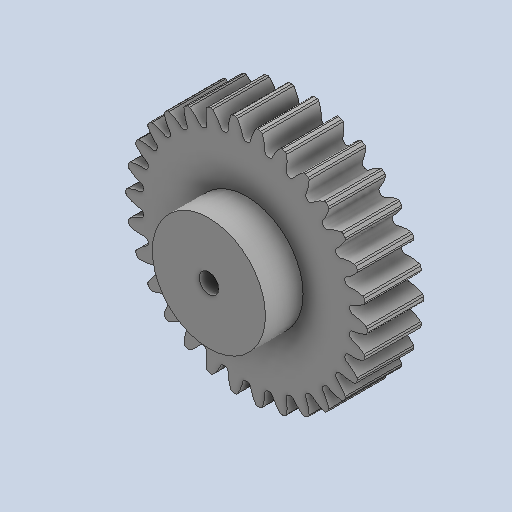
# Autodesk Inventor part: input_gear_3
Saved by Autodesk Inventor 2024 (Build 280153000, 153)
## iProperties
Created: 2023-10-31
Part Number: input_gear_3
Material: Generic
Document SubType Name: Modeling
Designer: MATEO
Density: 1 g/cm^3
Appearance: Default
Mass: 48.8877 g
Surface Area: 121.627 cm^2
Volume: 48.8877 cm^3
Author: MATEO
Autodesk Inventor part; units mm, degrees
ref_plane "YZ Plane" through (0, 0, 0) normal (1, 0, 0) x (0, 1, 0)
ref_plane "XZ Plane" through (0, 0, 0) normal (0, 1, 0) x (-1, 0, 0)
ref_plane "XY Plane" through (0, 0, 0) normal (0, 0, 1) x (1, 0, 0)
sketch "Sketch1" plane through (0, 0, 0) normal (0, 0, 1) x (1, 0, 0)
  spline S0 degree 3 poles (-2.6104, 31.8934) (-2.4905, 31.7032) (-2.3108, 31.4181) (-2.0897, 31.0267) (-1.9309, 30.7294) (-1.7804, 30.4278) (-1.6387, 30.1219) (-1.5066, 29.8118) (-1.3852, 29.4973) (-1.2762, 29.1783) (-1.1803, 28.855) (-1.1178, 28.5811) (-1.0727, 28.361) (-1.025, 28.1991) (-0.9606, 28.0431) (-0.8767, 27.8964) (-0.7882, 27.7867) (-0.7083, 27.7075) (-0.6407, 27.657) (-0.5715, 27.6086) (-0.4953, 27.5725) (-0.4177, 27.539) (-0.3357, 27.5192) (-0.2529, 27.5025) (-0.1404, 27.4985) (0, 27.501) (0.1404, 27.4985) (0.2529, 27.5025) (0.3357, 27.5192) (0.4177, 27.539) (0.4953, 27.5725) (0.5715, 27.6086) (0.6407, 27.657) (0.7083, 27.7075) (0.7882, 27.7867) (0.8767, 27.8964) (0.9606, 28.0431) (1.025, 28.1991) (1.0727, 28.361) (1.1178, 28.5811) (1.1803, 28.855) (1.2762, 29.1783) (1.3852, 29.4973) (1.5066, 29.8118) (1.6387, 30.1219) (1.7804, 30.4278) (1.9309, 30.7294) (2.0897, 31.0267) (2.3108, 31.4181) (2.4905, 31.7032) (2.6104, 31.8934) knots 0 0 0 0 0.067405 0.101109 0.134814 0.168518 0.202222 0.235926 0.26963 0.303333 0.337035 0.370735 0.387584 0.40443 0.421277 0.438116 0.454951 0.463377 0.471802 0.480225 0.488651 0.497074 0.505499 0.513923 0.522347 0.5392 0.556053 0.564477 0.572901 0.581327 0.589749 0.598176 0.606598 0.615023 0.623449 0.640284 0.657123 0.67397 0.690816 0.707665 0.741365 0.775067 0.80877 0.842474 0.876178 0.909882 0.943586 0.977291 1.010995 1.0784 1.0784 1.0784 1.0784
  circle A0 centre (0, 0) radius 27.5 construction
  circle A1 centre (0, 0) radius 28.1908 construction
  circle A2 centre (0, 0) radius 30
  circle A3 centre (0, 0) radius 32
  point P0 (-2.2571, 31.3193)
  point P1 (-2.0909, 31.0261)
  point P2 (-1.9323, 30.7287)
  point P3 (-1.7819, 30.4271)
  point P4 (-1.6403, 30.1212)
  point P5 (-1.5084, 29.811)
  point P6 (-1.3873, 29.4965)
  point P7 (-1.2784, 29.1776)
  point P8 (-1.1837, 28.8541)
  point P9 (-1.1069, 28.526)
  point P10 (-1.0704, 28.3615)
  point P11 (-1.0222, 28.2001)
  point P12 (-0.9574, 28.0446)
  point P13 (-0.873, 27.8989)
  point P14 (-0.7675, 27.7676)
  point P15 (-0.707, 27.709)
  point P16 (-0.6405, 27.6573)
  point P17 (-0.5704, 27.6107)
  point P18 (-0.495, 27.5729)
  point P19 (-0.417, 27.5413)
  point P20 (-0.3355, 27.5197)
  point P21 (-0.2526, 27.5047)
  point P22 (-0.1685, 27.5)
  point P23 (0, 27.5)
  point P24 (0.1685, 27.5)
  point P25 (0.2526, 27.5047)
  point P26 (0.3355, 27.5197)
  point P27 (0.417, 27.5413)
  point P28 (0.495, 27.5729)
  point P29 (0.5704, 27.6107)
  point P30 (0.6405, 27.6573)
  point P31 (0.707, 27.709)
  point P32 (0.7675, 27.7676)
  point P33 (0.873, 27.8989)
  point P34 (0.9574, 28.0446)
  point P35 (1.0222, 28.2001)
  point P36 (1.0704, 28.3615)
  point P37 (1.1069, 28.526)
  point P38 (1.1837, 28.8541)
  point P39 (1.2784, 29.1776)
  point P40 (1.3873, 29.4965)
  point P41 (1.5084, 29.811)
  point P42 (1.6403, 30.1212)
  point P43 (1.7819, 30.4271)
  point P44 (1.9323, 30.7287)
  point P45 (2.0909, 31.0261)
  point P46 (2.2571, 31.3193)
  constraints: 4 centre point, 2 point on circle, 103 other
extrude "Extrusion1" add sketch "Sketch1" against normal blind 15
surface extrude "ExtrusionSrf1" sketch "Sketch1" against normal through all shown no curves A2
extrude "Extrusion2" cut sketch "Sketch1" against normal through all contours A3 S0 A2 | A2 S0 picked at (0.1745, 31.3239) picked at (0.1505, 28.9695)
pattern_circular "Circular Pattern1" count 30 over 360 about axis through (0, 0, 0) along (0, 0, -1) of "Extrusion2"
sketch "Sketch2" plane through (0, 0, 0) normal (0, 0, 1) x (1, 0, 0)
  circle A0 centre (0, 0) radius 15
  circle A1 centre (0, 0) radius 2.6
  dimension "d7" = 30
  dimension "d8" = 5.2
  constraints: 2 centre point, 2 coincident
  measures "d7" diameter of A0
  measures "d8" diameter of A1
extrude "Extrusion3" add sketch "Sketch2" along normal blind 10
fillet "Fillet1" radius 0.5 2 edges at (4.0777, 31.7391, -7.5) (2.6104, 31.8934, -7.5)
pattern_circular "Circular Pattern2" count 30 over 360 about axis through (0, 0, 0) along (0, 0, 1) of "Fillet1"
extrude "Extrusion4" cut sketch "Sketch2" against normal through all contours A1
equation "\"Module\" = 2"
equation "\"PressureAngle\" = 20deg"
equation "\"UnitProfileClearance\" = 0.25"
equation "\"UnitRoundRadius\" = 0.35"
equation "\"HeadDiameter\" = 64"
equation "\"RootDiameter\" = 55"
equation "\"BaseDiameter\" = 56.38156"
equation "\"HelixAngle\" = 0"
equation "\"UnitCorrection\" = 0"
equation "\"UnitAddendumModification\" = 0"
equation "\"CircularPitch\" = 6.283185"
equation "\"UnitBacklashShift\" = 0"
equation "\"TotalToolShift\" = 0"
equation "\"IsInternal\" = 0"
body "Solid1"
body "Srf1"
